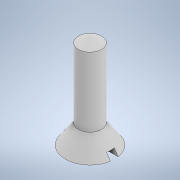
# Autodesk Inventor part: pieza7
Saved by Autodesk Inventor 2021 (Build 250183000, 183)
## iProperties
Created: 2020-10-13
Part Number: pieza7
Material: Generic
Document SubType Name: Modeling
Designer: carlo
Density: 1 g/cm^3
Appearance: Default
Author: carlo
Autodesk Inventor part; units mm, degrees
ref_plane "YZ Plane" through (0, 0, 0) normal (1, 0, 0) x (0, 1, 0)
sketch "Sketch1" plane through (0, 0, 0) normal (0, 1, 0) x (-1, 0, 0)
  circle A0 centre (0, 0) radius 6.385
  dimension "d0" = 12.77
  constraints: 1 centre point, 1 coincident
  measures "d0" diameter of A0
ref_plane "Work Plane1" through (0, 5, 0) normal (0, 1, 0) x (-1, 0, 0)
sketch "Sketch2" plane through (0, 5, 0) normal (0, 1, 0) x (-1, 0, 0)
  circle A0 centre (0, 0) radius 3
  dimension "d2" = 6
  constraints: 1 centre point, 1 coincident
  measures "d2" diameter of A0
extrude "Extrusion1" add sketch "Sketch2" along normal blind 18
loft "Loft1" add profiles "Sketch1" section 2 edges at (3, 5, 0)
sketch "Sketch3" plane through (0, 0, 0) normal (1, 0, 0) x (0, 1, 0)
  line L0 (1.5, 1) -> (-1.5, 1)
  line L1 (-1.5, 1) -> (-1.5, -1)
  line L2 (-1.5, -1) -> (1.5, -1)
  line L3 (1.5, -1) -> (1.5, 1)
  line L4 (1.5, 1) -> (-1.5, -1) construction
  line L5 (-1.5, 1) -> (1.5, -1) construction
  point P0 (0, 0)
  dimension "d9" = 3
  dimension "d10" = 2
  constraints: 12 end point, 2 midpoint, 2 parallel, 1 horizontal, 1 perpendicular
  measures "d9" distance of L2.end L1.end
  measures "d10" distance of L1.end L0.end
extrude "Extrusion2" cut sketch "Sketch3" along normal mid plane 15
sketch "Sketch5" plane through (0, 0, 0) normal (1, 0, 0) x (0, 1, 0)
  line L0 (23, -3) -> (23, 3) projected
  line L1 (23, 3) -> (24.7321, 0)
  line L2 (24.7321, 0) -> (23, -3)
  line L3 (23, -3) -> (23, 3)
  point P0 (0, 0)
  dimension "d13" = 120
  constraints: 6 end point, 1 equal length, 1 vertical
  measures "d13" angle of L1 L2
sketch "Sketch8" plane through (0, 0, 0) normal (1, 0, 0) x (0, 1, 0)
  point P0 (0, 0)
ref_plane "Work Plane2" through (0, 24.732, 0) normal (0, 1, 0) x (1, 0, 0)
sketch "Sketch9" plane through (0, 24.732, 0) normal (0, 1, 0) x (1, 0, 0)
  circle A0 centre (0, 0) radius 0.0005
  dimension "d15" = 0.001
  constraints: 1 centre point, 1 coincident
  measures "d15" diameter of A0
loft "Loft2" add profiles "Sketch9" section 1 edges at (3, 23, 0)
body "Solid1"
